Autodesk Inventor part; units mm, degrees
(part 3 of 4)
sketch "Эскиз8" plane through (0, 0, 5) normal (0, 0, 1) x (1, 0, 0)
  line L0 (-3.3401, -49.353) -> (-3.9955, -49.0011) projected
  line L1 (-3.9955, -49.0011) -> (-4.6711, -48.6896) projected
  line L2 (-4.6711, -48.6896) -> (-4.9594, -48.4736) projected
  line L3 (-4.9594, -48.4736) -> (-5.0531, -48.3399) projected
  line L4 (-5.0531, -48.3399) -> (-5.1131, -48.2201) projected
  line L5 (-5.1131, -48.2201) -> (-5.1548, -48.1078) projected
  line L6 (-5.1548, -48.1078) -> (-5.1842, -48.0004) projected
  line L7 (-5.1842, -48.0004) -> (-5.2179, -47.7953) projected
  line L8 (-5.2179, -47.7953) -> (-5.2276, -47.5993) projected
  line L9 (-5.2276, -47.5993) -> (-5.2195, -47.4096) projected
  line L10 (-5.2195, -47.4096) -> (-5.1972, -47.225) projected
  line L11 (-5.1972, -47.225) -> (-5.1181, -46.8673) projected
  line L12 (-5.1181, -46.8673) -> (-5.0105, -46.5192) projected
  line L13 (-5.0105, -46.5192) -> (-4.963, -46.1513) projected
  line L14 (-4.963, -46.1513) -> (-4.956, -45.7709) projected
  line L15 (-4.956, -45.7709) -> (-4.9802, -45.3817) projected
  line L16 (-4.9802, -45.3817) -> (-5.0317, -44.9857) projected
  line L17 (-5.0317, -44.9857) -> (-5.1086, -44.5842) projected
  line L18 (-5.1086, -44.5842) -> (-5.2096, -44.1783) projected
  line L19 (-5.2096, -44.1783) -> (-5.3339, -43.7691) projected
  line L20 (-5.3339, -43.7691) -> (-5.4808, -43.3575) projected
  line L21 (-5.4808, -43.3575) -> (-5.65, -42.9443) projected
  line L22 (-5.65, -42.9443) -> (-5.7913, -42.6339) projected
  line L23 (-5.7913, -42.6339) -> (-7.9172, -42.3165) projected
  line L24 (-7.9172, -42.3165) -> (-8.143, -42.5721) projected
  line L25 (-8.143, -42.5721) -> (-8.4255, -42.9179) projected
  line L26 (-8.4255, -42.9179) -> (-8.6862, -43.2687) projected
  line L27 (-8.6862, -43.2687) -> (-8.9246, -43.6237) projected
  line L28 (-8.9246, -43.6237) -> (-9.1398, -43.9824) projected
  line L29 (-9.1398, -43.9824) -> (-9.3306, -44.3439) projected
  line L30 (-9.3306, -44.3439) -> (-9.4955, -44.7076) projected
  line L31 (-9.4955, -44.7076) -> (-9.6323, -45.0728) projected
  line L32 (-9.6323, -45.0728) -> (-9.7367, -45.4387) projected
  line L33 (-9.7367, -45.4387) -> (-9.7987, -45.8044) projected
  line L34 (-9.7987, -45.8044) -> (-9.7975, -46.1687) projected
  line L35 (-9.7975, -46.1687) -> (-9.8263, -46.5339) projected
  line L36 (-9.8263, -46.5339) -> (-9.8589, -46.717) projected
  line L37 (-9.8589, -46.717) -> (-9.9066, -46.9008) projected
  line L38 (-9.9066, -46.9008) -> (-9.9731, -47.0854) projected
  line L39 (-9.9731, -47.0854) -> (-10.0652, -47.2717) projected
  line L40 (-10.0652, -47.2717) -> (-10.1248, -47.3659) projected
  line L41 (-10.1248, -47.3659) -> (-10.1974, -47.4611) projected
  line L42 (-10.1974, -47.4611) -> (-10.2897, -47.5581) projected
  line L43 (-10.2897, -47.5581) -> (-10.4185, -47.6586) projected
  line L44 (-10.4185, -47.6586) -> (-10.7573, -47.781) projected
  line L45 (-10.7573, -47.781) -> (-11.4943, -47.8816) projected
  line L46 (-11.4943, -47.8816) -> (-12.2239, -48.0267) projected
  line L47 (-12.2239, -48.0267) -> (-12.5841, -48.0214) projected
  line L48 (-12.5841, -48.0214) -> (-12.7386, -47.9683) projected
  line L49 (-12.7386, -47.9683) -> (-12.8575, -47.9067) projected
  line L50 (-12.8575, -47.9067) -> (-12.9572, -47.8403) projected
  line L51 (-12.9572, -47.8403) -> (-13.0442, -47.7707) projected
  line L52 (-13.0442, -47.7707) -> (-13.192, -47.6246) projected
  line L53 (-13.192, -47.6246) -> (-13.3151, -47.4717) projected
  line L54 (-13.3151, -47.4717) -> (-13.42, -47.3135) projected
  line L55 (-13.42, -47.3135) -> (-13.5105, -47.151) projected
  line L56 (-13.5105, -47.151) -> (-13.6567, -46.8152) projected
  line L57 (-13.6567, -46.8152) -> (-13.7743, -46.4703) projected
  line L58 (-13.7743, -46.4703) -> (-13.9521, -46.1448) projected
  line L59 (-13.9521, -46.1448) -> (-14.17, -45.8329) projected
  line L60 (-14.17, -45.8329) -> (-14.4183, -45.5322) projected
  line L61 (-14.4183, -45.5322) -> (-14.6928, -45.2421) projected
  line L62 (-14.6928, -45.2421) -> (-14.991, -44.9625) projected
  line L63 (-14.991, -44.9625) -> (-15.3113, -44.6935) projected
  line L64 (-15.3113, -44.6935) -> (-15.6524, -44.4355) projected
  line L65 (-15.6524, -44.4355) -> (-16.0132, -44.1889) projected
  line L66 (-16.0132, -44.1889) -> (-16.3929, -43.954) projected
  line L67 (-16.3929, -43.954) -> (-16.6897, -43.7859) projected
  line L68 (-16.6897, -43.7859) -> (-18.5962, -44.7788) projected
  line L69 (-18.5962, -44.7788) -> (-18.6286, -45.1183) projected
  line L70 (-18.6286, -45.1183) -> (-18.6538, -45.564) projected
  line L71 (-18.6538, -45.564) -> (-18.6586, -46.0011) projected
  line L72 (-18.6586, -46.0011) -> (-18.6428, -46.4284) projected
  line L73 (-18.6428, -46.4284) -> (-18.606, -46.8451) projected
  line L74 (-18.606, -46.8451) -> (-18.5479, -47.2497) projected
  line L75 (-18.5479, -47.2497) -> (-18.4676, -47.6409) projected
  line L76 (-18.4676, -47.6409) -> (-18.3636, -48.0168) projected
  line L77 (-18.3636, -48.0168) -> (-18.233, -48.3741) projected
  line L78 (-18.233, -48.3741) -> (-18.0682, -48.7064) projected
  line L79 (-18.0682, -48.7064) -> (-17.8531, -49.0005) projected
  line L80 (-17.8531, -49.0005) -> (-17.6617, -49.3128) projected
  line L81 (-17.6617, -49.3128) -> (-17.5804, -49.4801) projected
  line L82 (-17.5804, -49.4801) -> (-17.511, -49.6568) projected
  line L83 (-17.511, -49.6568) -> (-17.4563, -49.8453) projected
  line L84 (-17.4563, -49.8453) -> (-17.4213, -50.0502) projected
  line L85 (-17.4213, -50.0502) -> (-17.4142, -50.1613) projected
  line L86 (-17.4142, -50.1613) -> (-17.417, -50.2811) projected
  line L87 (-17.417, -50.2811) -> (-17.4346, -50.4138) projected
  line L88 (-17.4346, -50.4138) -> (-17.4797, -50.5708) projected
  line L89 (-17.4797, -50.5708) -> (-17.6818, -50.869) projected
  line L90 (-17.6818, -50.869) -> (-18.219, -51.3836) projected
  line L91 (-18.219, -51.3836) -> (-18.724, -51.9298) projected
  line L92 (-18.724, -51.9298) -> (-19.0185, -52.1372) projected
  line L93 (-19.0185, -52.1372) -> (-19.1747, -52.1851) projected
  line L94 (-19.1747, -52.1851) -> (-19.3071, -52.2051) projected
  line L95 (-19.3071, -52.2051) -> (-19.4268, -52.2101) projected
  line L96 (-19.4268, -52.2101) -> (-19.5381, -52.2049) projected
  line L97 (-19.5381, -52.2049) -> (-19.7435, -52.1736) projected
  line L98 (-19.7435, -52.1736) -> (-19.933, -52.1222) projected
  line L99 (-19.933, -52.1222) -> (-20.1108, -52.0559) projected
  line L100 (-20.1108, -52.0559) -> (-20.2796, -51.9776) projected
  line L101 (-20.2796, -51.9776) -> (-20.5952, -51.7918) projected
  line L102 (-20.5952, -51.7918) -> (-20.8931, -51.5819) projected
  line L103 (-20.8931, -51.5819) -> (-21.2283, -51.4231) projected
  line L104 (-21.2283, -51.4231) -> (-21.5879, -51.2989) projected
  line L105 (-21.5879, -51.2989) -> (-21.9655, -51.2016) projected
  line L106 (-21.9655, -51.2016) -> (-22.3581, -51.1282) projected
  line L107 (-22.3581, -51.1282) -> (-22.7637, -51.0773) projected
  line L108 (-22.7637, -51.0773) -> (-23.1809, -51.0479) projected
  line L109 (-23.1809, -51.0479) -> (-23.6085, -51.0397) projected
  line L110 (-23.6085, -51.0397) -> (-24.0454, -51.0522) projected
  line L111 (-24.0454, -51.0522) -> (-24.4906, -51.0855) projected
  line L112 (-24.4906, -51.0855) -> (-24.8295, -51.1239) projected
  line L113 (-24.8295, -51.1239) -> (-25.7883, -53.0477) projected
  line L114 (-25.7883, -53.0477) -> (-25.615, -53.3414) projected
  line L115 (-25.615, -53.3414) -> (-25.3734, -53.7169) projected
  line L116 (-25.3734, -53.7169) -> (-25.1204, -54.0733) projected
  line L117 (-25.1204, -54.0733) -> (-24.8564, -54.4097) projected
  line L118 (-24.8564, -54.4097) -> (-24.5818, -54.7252) projected
  line L119 (-24.5818, -54.7252) -> (-24.2969, -55.0184) projected
  line L120 (-24.2969, -55.0184) -> (-24.0019, -55.2877) projected
  line L121 (-24.0019, -55.2877) -> (-23.6969, -55.5306) projected
  line L122 (-23.6969, -55.5306) -> (-23.3812, -55.7429) projected
  line L123 (-23.3812, -55.7429) -> (-23.0526, -55.9149) projected
  line L124 (-23.0526, -55.9149) -> (-22.7057, -56.0264) projected
  line L125 (-22.7057, -56.0264) -> (-22.3673, -56.1666) projected
  line L126 (-22.3673, -56.1666) -> (-22.2032, -56.2542) projected
  line L127 (-22.2032, -56.2542) -> (-22.0432, -56.3563) projected
  line L128 (-22.0432, -56.3563) -> (-21.8881, -56.4766) projected
  line L129 (-21.8881, -56.4766) -> (-21.7394, -56.6218) projected
  line L130 (-21.7394, -56.6218) -> (-21.6683, -56.7075) projected
  line L131 (-21.6683, -56.7075) -> (-21.6001, -56.806) projected
  line L132 (-21.6001, -56.806) -> (-21.5364, -56.9238) projected
  line L133 (-21.5364, -56.9238) -> (-21.4806, -57.0773) projected
  line L134 (-21.4806, -57.0773) -> (-21.4689, -57.4374) projected
  line L135 (-21.4689, -57.4374) -> (-21.601, -58.1694) projected
  line L136 (-21.601, -58.1694) -> (-21.6884, -58.9082) projected
  line L137 (-21.6884, -58.9082) -> (-21.8048, -59.2491) projected
  line L138 (-21.8048, -59.2491) -> (-21.903, -59.3796) projected
  line L139 (-21.903, -59.3796) -> (-21.9984, -59.4736) projected
  line L140 (-21.9984, -59.4736) -> (-22.0923, -59.548) projected
  line L141 (-22.0923, -59.548) -> (-22.1854, -59.6092) projected
  line L142 (-22.1854, -59.6092) -> (-22.37, -59.7046) projected
  line L143 (-22.37, -59.7046) -> (-22.5535, -59.7744) projected
  line L144 (-22.5535, -59.7744) -> (-22.7363, -59.8253) projected
  line L145 (-22.7363, -59.8253) -> (-22.9189, -59.8611) projected
  line L146 (-22.9189, -59.8611) -> (-23.2834, -59.8964) projected
  line L147 (-23.2834, -59.8964) -> (-23.6478, -59.9017) projected
  line L148 (-23.6478, -59.9017) -> (-24.0123, -59.9702) projected
  line L149 (-24.0123, -59.9702) -> (-24.3762, -60.0811) projected
  line L150 (-24.3762, -60.0811) -> (-24.7389, -60.2243) projected
  line L151 (-24.7389, -60.2243) -> (-25.0997, -60.3957) projected
  line L152 (-25.0997, -60.3957) -> (-25.4578, -60.5929) projected
  line L153 (-25.4578, -60.5929) -> (-25.8125, -60.8144) projected
  line L154 (-25.8125, -60.8144) -> (-26.1633, -61.0591) projected
  line L155 (-26.1633, -61.0591) -> (-26.5094, -61.326) projected
  line L156 (-26.5094, -61.326) -> (-26.8501, -61.6146) projected
  line L157 (-26.8501, -61.6146) -> (-27.1017, -61.8449) projected
  line L158 (-27.1017, -61.8449) -> (-26.7465, -63.9648) projected
  line L159 (-26.7465, -63.9648) -> (-26.4337, -64.1006) projected
  line L160 (-26.4337, -64.1006) -> (-26.0175, -64.2624) projected
  line L161 (-26.0175, -64.2624) -> (-25.6033, -64.402) projected
  line L162 (-25.6033, -64.402) -> (-25.192, -64.519) projected
  line L163 (-25.192, -64.519) -> (-24.7844, -64.6128) projected
  line L164 (-24.7844, -64.6128) -> (-24.3816, -64.6825) projected
  line L165 (-24.3816, -64.6825) -> (-23.9847, -64.727) projected
  line L166 (-23.9847, -64.727) -> (-23.5951, -64.7442) projected
  line L167 (-23.5951, -64.7442) -> (-23.2149, -64.7305) projected
  line L168 (-23.2149, -64.7305) -> (-22.848, -64.6765) projected
  line L169 (-22.848, -64.6765) -> (-22.5018, -64.5627) projected
  line L170 (-22.5018, -64.5627) -> (-22.1456, -64.4773) projected
  line L171 (-22.1456, -64.4773) -> (-21.9614, -64.4516) projected
  line L172 (-21.9614, -64.4516) -> (-21.7719, -64.4402) projected
  line L173 (-21.7719, -64.4402) -> (-21.5757, -64.4464) projected
  line L174 (-21.5757, -64.4464) -> (-21.3701, -64.4764) projected
  line L175 (-21.3701, -64.4764) -> (-21.2621, -64.504) projected
  line L176 (-21.2621, -64.504) -> (-21.1491, -64.5437) projected
  line L177 (-21.1491, -64.5437) -> (-21.0284, -64.6015) projected
  line L178 (-21.0284, -64.6015) -> (-20.8929, -64.6929) projected
  line L179 (-20.8929, -64.6929) -> (-20.6718, -64.9773) projected
  line L180 (-20.6718, -64.9773) -> (-20.3484, -65.6472) projected
  line L181 (-20.3484, -65.6472) -> (-19.985, -66.2962) projected
  circle A0 centre (-9.4677, -59.9808) radius 2.5 projected
  circle A1 centre (-2.274, -63.481) radius 1.6 projected
  circle A2 centre (-5.9675, -52.7871) radius 1.6 projected
  circle A3 centre (-16.6613, -56.4807) radius 1.6 projected
  circle A4 centre (-12.9678, -67.1745) radius 1.6 projected
  arc A5 (-27.2901, -112.9599) -> (-22.8404, -113.0615) centre (-25.0135, -110.7468) ccw projected
  line L182 (-25.0135, -110.7468) -> (-25.0135, -76.7468)
  line L183 (-25.0135, -110.7468) -> (8.9865, -110.7468) construction
  line L184 (-46.2049, -99.4426) -> (-29.9022, -115.8548)
  line L185 (-29.9022, -115.8548) -> (-56.6455, -115.6472)
  line L186 (-25.5981, -48.7632) -> (-26.9625, -47.1023) projected
  line L187 (-27.3014, -47.1406) -> (-26.9625, -47.1023) projected
  line L188 (-27.7429, -47.2077) -> (-27.3014, -47.1406) projected
  line L189 (-28.1715, -47.2931) -> (-27.7429, -47.2077) projected
  line L190 (-28.5864, -47.3967) -> (-28.1715, -47.2931) projected
  line L191 (-28.9865, -47.5185) -> (-28.5864, -47.3967) projected
  line L192 (-29.3705, -47.6588) -> (-28.9865, -47.5185) projected
  line L193 (-29.7368, -47.818) -> (-29.3705, -47.6588) projected
  line L194 (-30.0831, -47.9973) -> (-29.7368, -47.818) projected
  line L195 (-30.4059, -48.1987) -> (-30.0831, -47.9973) projected
  line L196 (-30.6971, -48.4284) -> (-30.4059, -48.1987) projected
  line L197 (-30.9405, -48.6995) -> (-30.6971, -48.4284) projected
  line L198 (-31.2067, -48.9511) -> (-30.9405, -48.6995) projected
  line L199 (-31.3536, -49.0652) -> (-31.2067, -48.9511) projected
  line L200 (-31.5122, -49.1695) -> (-31.3536, -49.0652) projected
  line L201 (-31.6854, -49.262) -> (-31.5122, -49.1695) projected
  line L202 (-31.8786, -49.3384) -> (-31.6854, -49.262) projected
  line L203 (-31.986, -49.3683) -> (-31.8786, -49.3384) projected
  line L204 (-32.1037, -49.3902) -> (-31.986, -49.3683) projected
  line L205 (-32.2372, -49.4003) -> (-32.1037, -49.3902) projected
  line L206 (-32.4002, -49.3886) -> (-32.2372, -49.4003) projected
  line L207 (-32.7336, -49.2522) -> (-32.4002, -49.3886) projected
  line L208 (-33.3479, -48.8326) -> (-32.7336, -49.2522) projected
  line L209 (-33.9864, -48.4511) -> (-33.3479, -48.8326) projected
  line L210 (-34.2501, -48.2056) -> (-33.9864, -48.4511) projected
  line L211 (-34.3291, -48.0626) -> (-34.2501, -48.2056) projected
  line L212 (-34.376, -47.9372) -> (-34.3291, -48.0626) projected
  line L213 (-34.4055, -47.8211) -> (-34.376, -47.9372) projected
  line L214 (-34.4234, -47.7112) -> (-34.4055, -47.8211) projected
  line L215 (-34.4351, -47.5037) -> (-34.4234, -47.7112) projected
  line L216 (-34.4238, -47.3077) -> (-34.4351, -47.5037) projected
  line L217 (-34.3956, -47.12) -> (-34.4238, -47.3077) projected
  line L218 (-34.3538, -46.9387) -> (-34.3956, -47.12) projected
  line L219 (-34.237, -46.5916) -> (-34.3538, -46.9387) projected
  line L220 (-34.0931, -46.2568) -> (-34.237, -46.5916) projected
  line L221 (-34.0067, -45.8961) -> (-34.0931, -46.2568) projected
  line L222 (-33.9593, -45.5186) -> (-34.0067, -45.8961) projected
  line L223 (-33.9419, -45.129) -> (-33.9593, -45.5186) projected
  line L224 (-33.951, -44.7298) -> (-33.9419, -45.129) projected
  line L225 (-33.9848, -44.3224) -> (-33.951, -44.7298) projected
  line L226 (-34.0421, -43.9081) -> (-33.9848, -44.3224) projected
  line L227 (-34.1221, -43.488) -> (-34.0421, -43.9081) projected
  line L228 (-34.2244, -43.063) -> (-34.1221, -43.488) projected
  line L229 (-34.3487, -42.6342) -> (-34.2244, -43.063) projected
  line L230 (-34.4561, -42.3105) -> (-34.3487, -42.6342) projected
  line L231 (-36.5363, -41.7688) -> (-34.4561, -42.3105) projected
  line L232 (-36.7879, -41.999) -> (-36.5363, -41.7688) projected
  line L233 (-37.1056, -42.3127) -> (-36.7879, -41.999) projected
  line L234 (-37.4022, -42.6338) -> (-37.1056, -42.3127) projected
  line L235 (-37.677, -42.9614) -> (-37.4022, -42.6338) projected
  line L236 (-37.9291, -43.2952) -> (-37.677, -42.9614) projected
  line L237 (-38.1573, -43.6344) -> (-37.9291, -43.2952) projected
  line L238 (-38.36, -43.9785) -> (-38.1573, -43.6344) projected
  line L239 (-38.5348, -44.327) -> (-38.36, -43.9785) projected
  line L240 (-38.6775, -44.6797) -> (-38.5348, -44.327) projected
  line L241 (-38.7781, -45.0367) -> (-38.6775, -44.6797) projected
  line L242 (-38.8157, -45.3992) -> (-38.7781, -45.0367) projected
  line L243 (-38.8831, -45.7592) -> (-38.8157, -45.3992) projected
  line L244 (-38.935, -45.9378) -> (-38.8831, -45.7592) projected
  line L245 (-39.0019, -46.1155) -> (-38.935, -45.9378) projected
  line L246 (-39.0877, -46.292) -> (-39.0019, -46.1155) projected
  line L247 (-39.1991, -46.4674) -> (-39.0877, -46.292) projected
  line L248 (-39.2684, -46.5547) -> (-39.1991, -46.4674) projected
  line L249 (-39.3507, -46.6417) -> (-39.2684, -46.5547) projected
  line L250 (-39.4528, -46.7283) -> (-39.3507, -46.6417) projected
  line L251 (-39.5916, -46.8146) -> (-39.4528, -46.7283) projected
  line L252 (-39.9414, -46.9002) -> (-39.5916, -46.8146) projected
  line L253 (-40.685, -46.9219) -> (-39.9414, -46.9002) projected
  line L254 (-41.4259, -46.9885) -> (-40.685, -46.9219) projected
  line L255 (-41.7835, -46.9449) -> (-41.4259, -46.9885) projected
  line L256 (-41.9315, -46.8757) -> (-41.7835, -46.9449) projected
  line L257 (-42.0431, -46.8018) -> (-41.9315, -46.8757) projected
  line L258 (-42.1352, -46.7252) -> (-42.0431, -46.8018) projected
  line L259 (-42.2143, -46.6467) -> (-42.1352, -46.7252) projected
  line L260 (-42.3457, -46.4857) -> (-42.2143, -46.6467) projected
  line L261 (-42.4518, -46.3206) -> (-42.3457, -46.4857) projected
  line L262 (-42.5394, -46.1522) -> (-42.4518, -46.3206) projected
  line L263 (-42.612, -45.9809) -> (-42.5394, -46.1522) projected
  line L264 (-42.7217, -45.6314) -> (-42.612, -45.9809) projected
  line L265 (-42.8019, -45.276) -> (-42.7217, -45.6314) projected
  line L266 (-42.9441, -44.9334) -> (-42.8019, -45.276) projected
  line L267 (-43.1276, -44.6002) -> (-42.9441, -44.9334) projected
  line L268 (-43.3425, -44.2748) -> (-43.1276, -44.6002) projected
  line L269 (-43.5846, -43.9571) -> (-43.3425, -44.2748) projected
  line L270 (-43.8514, -43.6473) -> (-43.5846, -43.9571) projected
  line L271 (-44.1412, -43.3458) -> (-43.8514, -43.6473) projected
  line L272 (-44.4529, -43.053) -> (-44.1412, -43.3458) projected
  line L273 (-44.5941, -42.9326) -> (-44.4529, -43.053) projected
  arc A6 (-44.5941, -42.9326) -> (-50.5827, -73.1948) centre (-31.1137, -61.3239) ccw projected
  arc A7 (-46.3063, -82.796) -> (-50.5827, -73.1948) centre (-85.5886, -94.5392) ccw projected
  line L274 (-46.3063, -82.796) -> (-63.0717, -107.6742) projected
  line L275 (-63.0717, -107.6742) -> (-48.9946, -134.1664) projected
  line L276 (-48.9946, -134.1664) -> (-45.4623, -132.2894) projected
  line L277 (-45.4623, -132.2894) -> (-58.0098, -108.6759) projected
  line L278 (-58.0098, -108.6759) -> (-41.2444, -83.7977) projected
  line L279 (-26.1708, -65.5638) -> (-41.2444, -83.7977) projected
  line L280 (-26.1708, -65.5638) -> (-26.1132, -65.2728) projected
  line L281 (-26.2817, -65.1065) -> (-26.1132, -65.2728) projected
  line L282 (-26.573, -64.8618) -> (-26.2817, -65.1065) projected
  line L283 (-26.8814, -64.6558) -> (-26.573, -64.8618) projected
  line L284 (-27.2145, -64.5081) -> (-26.8814, -64.6558) projected
  line L285 (-27.5361, -64.3327) -> (-27.2145, -64.5081) projected
  line L286 (-27.6899, -64.2282) -> (-27.5361, -64.3327) projected
  line L287 (-27.8382, -64.1096) -> (-27.6899, -64.2282) projected
  line L288 (-27.9796, -63.9735) -> (-27.8382, -64.1096) projected
  line L289 (-28.112, -63.8133) -> (-27.9796, -63.9735) projected
  line L290 (-28.1736, -63.7205) -> (-28.112, -63.8133) projected
  line L291 (-28.2309, -63.6153) -> (-28.1736, -63.7205) projected
  line L292 (-28.2817, -63.4914) -> (-28.2309, -63.6153) projected
  line L293 (-28.3209, -63.3328) -> (-28.2817, -63.4914) projected
  line L294 (-28.2942, -62.9735) -> (-28.3209, -63.3328) projected
  line L295 (-28.085, -62.2597) -> (-28.2942, -62.9735) projected
  line L296 (-27.9195, -61.5344) -> (-28.085, -62.2597) projected
  line L297 (-27.7675, -61.2078) -> (-27.9195, -61.5344) projected
  line L298 (-27.6559, -61.0885) -> (-27.7675, -61.2078) projected
  line L299 (-27.5511, -61.0052) -> (-27.6559, -61.0885) projected
  line L300 (-27.4498, -60.9413) -> (-27.5511, -61.0052) projected
  line L301 (-27.3508, -60.8903) -> (-27.4498, -60.9413) projected
  line L302 (-27.1571, -60.815) -> (-27.3508, -60.8903) projected
  line L303 (-26.9672, -60.7651) -> (-27.1571, -60.815) projected
  line L304 (-26.78, -60.734) -> (-26.9672, -60.7651) projected
  line L305 (-26.5947, -60.7178) -> (-26.78, -60.734) projected
  line L306 (-26.2284, -60.7215) -> (-26.5947, -60.7178) projected
  line L307 (-25.8656, -60.755) -> (-26.2284, -60.7215) projected
  line L308 (-25.4958, -60.7256) -> (-25.8656, -60.755) projected
  line L309 (-25.1221, -60.6541) -> (-25.4958, -60.7256) projected
  line L310 (-24.7463, -60.5502) -> (-25.1221, -60.6541) projected
  line L311 (-24.3693, -60.4182) -> (-24.7463, -60.5502) projected
  line L312 (-23.9923, -60.2602) -> (-24.3693, -60.4182) projected
  line L313 (-23.616, -60.0777) -> (-23.9923, -60.2602) projected
  line L314 (-23.2412, -59.8717) -> (-23.616, -60.0777) projected
  line L315 (-22.8687, -59.6431) -> (-23.2412, -59.8717) projected
  line L316 (-22.4992, -59.3924) -> (-22.8687, -59.6431) projected
  line L317 (-22.2246, -59.1902) -> (-22.4992, -59.3924) projected
  line L318 (-22.3522, -57.0445) -> (-22.2246, -59.1902) projected
  line L319 (-22.6489, -56.8763) -> (-22.3522, -57.0445) projected
  line L320 (-23.0454, -56.6711) -> (-22.6489, -56.8763) projected
  line L321 (-23.4424, -56.4882) -> (-23.0454, -56.6711) projected
  line L322 (-23.839, -56.3281) -> (-23.4424, -56.4882) projected
  line L323 (-24.2343, -56.1915) -> (-23.839, -56.3281) projected
  line L324 (-24.6274, -56.0793) -> (-24.2343, -56.1915) projected
  line L325 (-25.0173, -55.9929) -> (-24.6274, -56.0793) projected
  line L326 (-25.4028, -55.9343) -> (-25.0173, -55.9929) projected
  line L327 (-25.7823, -55.9075) -> (-25.4028, -55.9343) projected
  line L328 (-26.153, -55.9222) -> (-25.7823, -55.9075) projected
  line L329 (-26.5093, -55.9985) -> (-26.153, -55.9222) projected
  line L330 (-26.8725, -56.0456) -> (-26.5093, -55.9985) projected
  line L331 (-27.0584, -56.0515) -> (-26.8725, -56.0456) projected
  line L332 (-27.248, -56.0427) -> (-27.0584, -56.0515) projected
  line L333 (-27.4425, -56.0157) -> (-27.248, -56.0427) projected
  line L334 (-27.6437, -55.9639) -> (-27.4425, -56.0157) projected
  line L335 (-27.7481, -55.925) -> (-27.6437, -55.9639) projected
  line L336 (-27.8563, -55.8736) -> (-27.7481, -55.925) projected
  line L337 (-27.9702, -55.8032) -> (-27.8563, -55.8736) projected
  line L338 (-28.0951, -55.698) -> (-27.9702, -55.8032) projected
  line L339 (-28.2847, -55.3917) -> (-28.0951, -55.698) projected
  line L340 (-28.5351, -54.6912) -> (-28.2847, -55.3917) projected
  line L341 (-28.8274, -54.0071) -> (-28.5351, -54.6912) projected
  line L342 (-28.8965, -53.6536) -> (-28.8274, -54.0071) projected
  line L343 (-28.8763, -53.4914) -> (-28.8965, -53.6536) projected
  line L344 (-28.8405, -53.3624) -> (-28.8763, -53.4914) projected
  line L345 (-28.7962, -53.2512) -> (-28.8405, -53.3624) projected
  line L346 (-28.746, -53.1517) -> (-28.7962, -53.2512) projected
  line L347 (-28.6335, -52.977) -> (-28.746, -53.1517) projected
  line L348 (-28.5092, -52.825) -> (-28.6335, -52.977) projected
  line L349 (-28.3761, -52.6897) -> (-28.5092, -52.825) projected
  line L350 (-28.2357, -52.5677) -> (-28.3761, -52.6897) projected
  line L351 (-27.9372, -52.3554) -> (-28.2357, -52.5677) projected
  line L352 (-27.624, -52.1693) -> (-27.9372, -52.3554) projected
  line L353 (-27.3421, -51.9282) -> (-27.624, -52.1693) projected
  line L354 (-27.0818, -51.6507) -> (-27.3421, -51.9282) projected
  line L355 (-26.8388, -51.3457) -> (-27.0818, -51.6507) projected
  line L356 (-26.6114, -51.0173) -> (-26.8388, -51.3457) projected
  line L357 (-26.3993, -50.6679) -> (-26.6114, -51.0173) projected
  line L358 (-26.2021, -50.2991) -> (-26.3993, -50.6679) projected
  line L359 (-26.02, -49.9121) -> (-26.2021, -50.2991) projected
  line L360 (-25.853, -49.5082) -> (-26.02, -49.9121) projected
  line L361 (-25.7014, -49.0882) -> (-25.853, -49.5082) projected
  line L362 (-25.5981, -48.7632) -> (-25.7014, -49.0882) projected
  circle A8 centre (-42.8052, -51.6922) radius 1.6 projected
  circle A9 centre (-39.9568, -59.168) radius 2.5 projected
  circle A10 centre (-32.4811, -56.3196) radius 1.6 projected
  circle A11 centre (-37.1084, -66.6437) radius 1.6 projected
  circle A12 centre (-47.4326, -62.0164) radius 1.6 projected
  line L363 (-46.3063, -82.796) -> (-41.3132, -83.8997)
  line L364 (-46.2049, -99.4426) -> (-41.3132, -83.8997)
  line L365 (-46.3063, -82.796) -> (-56.6455, -115.6472)
  arc A13 (-19.985, -66.2962) -> (-3.3401, -49.353) centre (-9.4677, -59.9808) ccw projected
  point P0 (0, 0)
  point P1 (-42.8913, -102.7785)
  point P2 (-56.6509, -115.6472)
  point P3 (-55.7751, -112.8815)
  point P4 (-54.2957, -115.6655)
  dimension "d21" = 34
  dimension "d22" = 90
  constraints: 14 end point, 3 point on line, 1 horizontal, 1 parallel, 1 perpendicular, 1 vertical
  measures "d21" distance of L182.start L182.end
  measures "d22" angle of L183 L182
extrude "Выдавливание8" add sketch "Эскиз8" against normal up to surface (5 mm away) contours L364 L184 L185 L277 L365 L278 | L278 L365 L363
sketch "Эскиз9" plane through (0, 0, 5) normal (0, 0, 1) x (1, 0, 0)
  line L0 (-41.3132, -83.8997) -> (-41.2444, -83.7977) projected
  line L1 (-26.1708, -65.5638) -> (-41.2444, -83.7977) projected
  line L2 (-26.1708, -65.5638) -> (-26.1132, -65.2728) projected
  line L3 (-26.2817, -65.1065) -> (-26.1132, -65.2728) projected
  line L4 (-26.573, -64.8618) -> (-26.2817, -65.1065) projected
  line L5 (-26.8814, -64.6558) -> (-26.573, -64.8618) projected
  line L6 (-27.2145, -64.5081) -> (-26.8814, -64.6558) projected
  line L7 (-27.5361, -64.3327) -> (-27.2145, -64.5081) projected
  line L8 (-27.6899, -64.2282) -> (-27.5361, -64.3327) projected
  line L9 (-27.8382, -64.1096) -> (-27.6899, -64.2282) projected
  line L10 (-27.9796, -63.9735) -> (-27.8382, -64.1096) projected
  line L11 (-28.112, -63.8133) -> (-27.9796, -63.9735) projected
  line L12 (-28.1736, -63.7205) -> (-28.112, -63.8133) projected
  line L13 (-28.2309, -63.6153) -> (-28.1736, -63.7205) projected
  line L14 (-28.2817, -63.4914) -> (-28.2309, -63.6153) projected
  line L15 (-28.3209, -63.3328) -> (-28.2817, -63.4914) projected
  line L16 (-28.2942, -62.9735) -> (-28.3209, -63.3328) projected
  line L17 (-28.085, -62.2597) -> (-28.2942, -62.9735) projected
  line L18 (-27.9195, -61.5344) -> (-28.085, -62.2597) projected
  line L19 (-27.7675, -61.2078) -> (-27.9195, -61.5344) projected
  line L20 (-27.6559, -61.0885) -> (-27.7675, -61.2078) projected
  line L21 (-27.5511, -61.0052) -> (-27.6559, -61.0885) projected
  line L22 (-27.4498, -60.9413) -> (-27.5511, -61.0052) projected
  line L23 (-27.3508, -60.8903) -> (-27.4498, -60.9413) projected
  line L24 (-27.1571, -60.815) -> (-27.3508, -60.8903) projected
  line L25 (-26.9672, -60.7651) -> (-27.1571, -60.815) projected
  line L26 (-26.78, -60.734) -> (-26.9672, -60.7651) projected
  line L27 (-26.5947, -60.7178) -> (-26.78, -60.734) projected
  line L28 (-26.2284, -60.7215) -> (-26.5947, -60.7178) projected
  line L29 (-25.8656, -60.755) -> (-26.2284, -60.7215) projected
  line L30 (-25.4958, -60.7256) -> (-25.8656, -60.755) projected
  line L31 (-25.1221, -60.6541) -> (-25.4958, -60.7256) projected
  line L32 (-24.7463, -60.5502) -> (-25.1221, -60.6541) projected
  line L33 (-24.3693, -60.4182) -> (-24.7463, -60.5502) projected
  line L34 (-23.9923, -60.2602) -> (-24.3693, -60.4182) projected
  line L35 (-23.616, -60.0777) -> (-23.9923, -60.2602) projected
  line L36 (-23.2412, -59.8717) -> (-23.616, -60.0777) projected
  line L37 (-22.8687, -59.6431) -> (-23.2412, -59.8717) projected
  line L38 (-22.4992, -59.3924) -> (-22.8687, -59.6431) projected
  line L39 (-22.2246, -59.1902) -> (-22.4992, -59.3924) projected
  line L40 (-22.3522, -57.0445) -> (-22.2246, -59.1902) projected
  line L41 (-22.6489, -56.8763) -> (-22.3522, -57.0445) projected
  line L42 (-23.0454, -56.6711) -> (-22.6489, -56.8763) projected
  line L43 (-23.4424, -56.4882) -> (-23.0454, -56.6711) projected
  line L44 (-23.839, -56.3281) -> (-23.4424, -56.4882) projected
  line L45 (-24.2343, -56.1915) -> (-23.839, -56.3281) projected
  line L46 (-24.6274, -56.0793) -> (-24.2343, -56.1915) projected
  line L47 (-25.0173, -55.9929) -> (-24.6274, -56.0793) projected
  line L48 (-25.4028, -55.9343) -> (-25.0173, -55.9929) projected
  line L49 (-25.7823, -55.9075) -> (-25.4028, -55.9343) projected
  line L50 (-26.153, -55.9222) -> (-25.7823, -55.9075) projected
  line L51 (-26.5093, -55.9985) -> (-26.153, -55.9222) projected
  line L52 (-26.8725, -56.0456) -> (-26.5093, -55.9985) projected
  line L53 (-27.0584, -56.0515) -> (-26.8725, -56.0456) projected
  line L54 (-27.248, -56.0427) -> (-27.0584, -56.0515) projected
  line L55 (-27.4425, -56.0157) -> (-27.248, -56.0427) projected
  line L56 (-27.6437, -55.9639) -> (-27.4425, -56.0157) projected
  line L57 (-27.7481, -55.925) -> (-27.6437, -55.9639) projected
  line L58 (-27.8563, -55.8736) -> (-27.7481, -55.925) projected
  line L59 (-27.9702, -55.8032) -> (-27.8563, -55.8736) projected
  line L60 (-28.0951, -55.698) -> (-27.9702, -55.8032) projected
  line L61 (-28.2847, -55.3917) -> (-28.0951, -55.698) projected
  line L62 (-28.5351, -54.6912) -> (-28.2847, -55.3917) projected
  line L63 (-28.8274, -54.0071) -> (-28.5351, -54.6912) projected
  line L64 (-28.8965, -53.6536) -> (-28.8274, -54.0071) projected
  line L65 (-28.8763, -53.4914) -> (-28.8965, -53.6536) projected
  line L66 (-28.8405, -53.3624) -> (-28.8763, -53.4914) projected
  line L67 (-28.7962, -53.2512) -> (-28.8405, -53.3624) projected
  line L68 (-28.746, -53.1517) -> (-28.7962, -53.2512) projected
  line L69 (-28.6335, -52.977) -> (-28.746, -53.1517) projected
  line L70 (-28.5092, -52.825) -> (-28.6335, -52.977) projected
  line L71 (-28.3761, -52.6897) -> (-28.5092, -52.825) projected
  line L72 (-28.2357, -52.5677) -> (-28.3761, -52.6897) projected
  line L73 (-27.9372, -52.3554) -> (-28.2357, -52.5677) projected
  line L74 (-27.624, -52.1693) -> (-27.9372, -52.3554) projected
  line L75 (-27.3421, -51.9282) -> (-27.624, -52.1693) projected
  line L76 (-27.0818, -51.6507) -> (-27.3421, -51.9282) projected
  line L77 (-26.8388, -51.3457) -> (-27.0818, -51.6507) projected
  line L78 (-26.6114, -51.0173) -> (-26.8388, -51.3457) projected
  line L79 (-26.3993, -50.6679) -> (-26.6114, -51.0173) projected
  line L80 (-26.2021, -50.2991) -> (-26.3993, -50.6679) projected
  line L81 (-26.02, -49.9121) -> (-26.2021, -50.2991) projected
  line L82 (-25.853, -49.5082) -> (-26.02, -49.9121) projected
  line L83 (-25.7014, -49.0882) -> (-25.853, -49.5082) projected
  line L84 (-25.5981, -48.7632) -> (-25.7014, -49.0882) projected
  line L85 (-25.5981, -48.7632) -> (-26.9625, -47.1023) projected
  line L86 (-27.3014, -47.1406) -> (-26.9625, -47.1023) projected
  line L87 (-27.7429, -47.2077) -> (-27.3014, -47.1406) projected
  line L88 (-28.1715, -47.2931) -> (-27.7429, -47.2077) projected
  line L89 (-28.5864, -47.3967) -> (-28.1715, -47.2931) projected
  line L90 (-28.9865, -47.5185) -> (-28.5864, -47.3967) projected
  line L91 (-29.3705, -47.6588) -> (-28.9865, -47.5185) projected
  line L92 (-29.7368, -47.818) -> (-29.3705, -47.6588) projected
  line L93 (-30.0831, -47.9973) -> (-29.7368, -47.818) projected
  line L94 (-30.4059, -48.1987) -> (-30.0831, -47.9973) projected
  line L95 (-30.6971, -48.4284) -> (-30.4059, -48.1987) projected
  line L96 (-30.9405, -48.6995) -> (-30.6971, -48.4284) projected
  line L97 (-31.2067, -48.9511) -> (-30.9405, -48.6995) projected
  line L98 (-31.3536, -49.0652) -> (-31.2067, -48.9511) projected
  line L99 (-31.5122, -49.1695) -> (-31.3536, -49.0652) projected
  line L100 (-31.6854, -49.262) -> (-31.5122, -49.1695) projected
  line L101 (-31.8786, -49.3384) -> (-31.6854, -49.262) projected
  line L102 (-31.986, -49.3683) -> (-31.8786, -49.3384) projected
  line L103 (-32.1037, -49.3902) -> (-31.986, -49.3683) projected
  line L104 (-32.2372, -49.4003) -> (-32.1037, -49.3902) projected
  line L105 (-32.4002, -49.3886) -> (-32.2372, -49.4003) projected
  line L106 (-32.7336, -49.2522) -> (-32.4002, -49.3886) projected
  line L107 (-33.3479, -48.8326) -> (-32.7336, -49.2522) projected
  line L108 (-33.9864, -48.4511) -> (-33.3479, -48.8326) projected
  line L109 (-34.2501, -48.2056) -> (-33.9864, -48.4511) projected
  line L110 (-34.3291, -48.0626) -> (-34.2501, -48.2056) projected
  line L111 (-34.376, -47.9372) -> (-34.3291, -48.0626) projected
  line L112 (-34.4055, -47.8211) -> (-34.376, -47.9372) projected
  line L113 (-34.4234, -47.7112) -> (-34.4055, -47.8211) projected
  line L114 (-34.4351, -47.5037) -> (-34.4234, -47.7112) projected
  line L115 (-34.4238, -47.3077) -> (-34.4351, -47.5037) projected
  line L116 (-34.3956, -47.12) -> (-34.4238, -47.3077) projected
  line L117 (-34.3538, -46.9387) -> (-34.3956, -47.12) projected
  line L118 (-34.237, -46.5916) -> (-34.3538, -46.9387) projected
  line L119 (-34.0931, -46.2568) -> (-34.237, -46.5916) projected
  line L120 (-34.0067, -45.8961) -> (-34.0931, -46.2568) projected
  line L121 (-33.9593, -45.5186) -> (-34.0067, -45.8961) projected
  line L122 (-33.9419, -45.129) -> (-33.9593, -45.5186) projected
  line L123 (-33.951, -44.7298) -> (-33.9419, -45.129) projected
  line L124 (-33.9848, -44.3224) -> (-33.951, -44.7298) projected
  line L125 (-34.0421, -43.9081) -> (-33.9848, -44.3224) projected
  line L126 (-34.1221, -43.488) -> (-34.0421, -43.9081) projected
  line L127 (-34.2244, -43.063) -> (-34.1221, -43.488) projected
  line L128 (-34.3487, -42.6342) -> (-34.2244, -43.063) projected
  line L129 (-34.4561, -42.3105) -> (-34.3487, -42.6342) projected
  line L130 (-36.5363, -41.7688) -> (-34.4561, -42.3105) projected
  line L131 (-36.7879, -41.999) -> (-36.5363, -41.7688) projected
  line L132 (-37.1056, -42.3127) -> (-36.7879, -41.999) projected
  line L133 (-37.4022, -42.6338) -> (-37.1056, -42.3127) projected
  line L134 (-37.677, -42.9614) -> (-37.4022, -42.6338) projected
  line L135 (-37.9291, -43.2952) -> (-37.677, -42.9614) projected
  line L136 (-38.1573, -43.6344) -> (-37.9291, -43.2952) projected
  line L137 (-38.36, -43.9785) -> (-38.1573, -43.6344) projected
  line L138 (-38.5348, -44.327) -> (-38.36, -43.9785) projected
  line L139 (-38.6775, -44.6797) -> (-38.5348, -44.327) projected
  line L140 (-38.7781, -45.0367) -> (-38.6775, -44.6797) projected
  line L141 (-38.8157, -45.3992) -> (-38.7781, -45.0367) projected
  line L142 (-38.8831, -45.7592) -> (-38.8157, -45.3992) projected
  line L143 (-38.935, -45.9378) -> (-38.8831, -45.7592) projected
  line L144 (-39.0019, -46.1155) -> (-38.935, -45.9378) projected
  line L145 (-39.0877, -46.292) -> (-39.0019, -46.1155) projected
  line L146 (-39.1991, -46.4674) -> (-39.0877, -46.292) projected
  line L147 (-39.2684, -46.5547) -> (-39.1991, -46.4674) projected
  line L148 (-39.3507, -46.6417) -> (-39.2684, -46.5547) projected
  line L149 (-39.4528, -46.7283) -> (-39.3507, -46.6417) projected
  line L150 (-39.5916, -46.8146) -> (-39.4528, -46.7283) projected
  line L151 (-39.9414, -46.9002) -> (-39.5916, -46.8146) projected
  line L152 (-40.685, -46.9219) -> (-39.9414, -46.9002) projected
  line L153 (-41.4259, -46.9885) -> (-40.685, -46.9219) projected
  line L154 (-41.7835, -46.9449) -> (-41.4259, -46.9885) projected
  line L155 (-41.9315, -46.8757) -> (-41.7835, -46.9449) projected
  line L156 (-42.0431, -46.8018) -> (-41.9315, -46.8757) projected
  line L157 (-42.1352, -46.7252) -> (-42.0431, -46.8018) projected
  line L158 (-42.2143, -46.6467) -> (-42.1352, -46.7252) projected
  line L159 (-42.3457, -46.4857) -> (-42.2143, -46.6467) projected
  line L160 (-42.4518, -46.3206) -> (-42.3457, -46.4857) projected
  line L161 (-42.5394, -46.1522) -> (-42.4518, -46.3206) projected
  line L162 (-42.612, -45.9809) -> (-42.5394, -46.1522) projected
  line L163 (-42.7217, -45.6314) -> (-42.612, -45.9809) projected
  line L164 (-42.8019, -45.276) -> (-42.7217, -45.6314) projected
  line L165 (-42.9441, -44.9334) -> (-42.8019, -45.276) projected
  line L166 (-43.1276, -44.6002) -> (-42.9441, -44.9334) projected
  line L167 (-43.3425, -44.2748) -> (-43.1276, -44.6002) projected
  line L168 (-43.5846, -43.9571) -> (-43.3425, -44.2748) projected
  line L169 (-43.8514, -43.6473) -> (-43.5846, -43.9571) projected
  line L170 (-44.1412, -43.3458) -> (-43.8514, -43.6473) projected
  line L171 (-44.4529, -43.053) -> (-44.1412, -43.3458) projected
  line L172 (-44.5941, -42.9326) -> (-44.4529, -43.053) projected
  arc A0 (-44.5941, -42.9326) -> (-50.5827, -73.1948) centre (-31.1137, -61.3239) ccw projected
  arc A1 (-46.3063, -82.796) -> (-50.5827, -73.1948) centre (-85.5886, -94.5392) ccw projected
  line L173 (-46.3063, -82.796) -> (-63.0717, -107.6742) projected
  line L174 (-63.0717, -107.6742) -> (-48.9946, -134.1664) projected
  line L175 (-48.9946, -134.1664) -> (-45.4623, -132.2894) projected
  line L176 (-45.4623, -132.2894) -> (-54.2957, -115.6655) projected
  line L177 (-54.2957, -115.6655) -> (-29.9022, -115.8548) projected
  line L178 (-29.9022, -115.8548) -> (-46.2049, -99.4426) projected
  line L179 (-46.2049, -99.4426) -> (-41.3132, -83.8997) projected
  circle A2 centre (-47.4326, -62.0164) radius 1.6 projected
  circle A3 centre (-37.1084, -66.6437) radius 1.6 projected
  circle A4 centre (-32.4811, -56.3196) radius 1.6 projected
  circle A5 centre (-39.9568, -59.168) radius 2.5 projected
  circle A6 centre (-42.8052, -51.6922) radius 1.6 projected
  line L180 (-51.3334, -98.7688) -> (-55.7751, -112.8815) projected
  line L181 (-55.7751, -112.8815) -> (-58.0098, -108.6759) projected
  line L182 (-58.0098, -108.6759) -> (-51.3334, -98.7688) projected
  line L183 (-51.3334, -98.7688) -> (-46.3063, -82.796)
  line L184 (-55.7751, -112.8815) -> (-55.7748, -115.6656)
  line L185 (-55.7748, -115.6656) -> (-54.2957, -115.6655)
  point P0 (0, 0)
  constraints: 6 end point, 1 perpendicular
extrude "Выдавливание9" cut sketch "Эскиз9" against normal through all contours L176 L175 L174 L173 L183 L182 L181 L184 L185
sketch "Эскиз10" plane through (0, 0, 5) normal (0, 0, 1) x (1, 0, 0)
  line L0 (-46.3063, -82.796) -> (-55.7751, -112.8815) projected
  line L1 (-55.7751, -112.8815) -> (-55.7748, -115.6656) projected
  line L2 (-55.7748, -115.6656) -> (-54.2957, -115.6655) projected
  line L3 (-54.2957, -115.6655) -> (-29.9022, -115.8548) projected
  line L4 (-29.9022, -115.8548) -> (-46.2049, -99.4426) projected
  line L5 (-46.2049, -99.4426) -> (-41.3132, -83.8997) projected
  line L6 (-41.3132, -83.8997) -> (-41.2444, -83.7977) projected
  line L7 (-26.1708, -65.5638) -> (-41.2444, -83.7977) projected
  line L8 (-26.1708, -65.5638) -> (-26.1132, -65.2728) projected
  line L9 (-26.2817, -65.1065) -> (-26.1132, -65.2728) projected
  line L10 (-26.573, -64.8618) -> (-26.2817, -65.1065) projected
  line L11 (-26.8814, -64.6558) -> (-26.573, -64.8618) projected
  line L12 (-27.2145, -64.5081) -> (-26.8814, -64.6558) projected
  line L13 (-27.5361, -64.3327) -> (-27.2145, -64.5081) projected
  line L14 (-27.6899, -64.2282) -> (-27.5361, -64.3327) projected
  line L15 (-27.8382, -64.1096) -> (-27.6899, -64.2282) projected
  line L16 (-27.9796, -63.9735) -> (-27.8382, -64.1096) projected
  line L17 (-28.112, -63.8133) -> (-27.9796, -63.9735) projected
  line L18 (-28.1736, -63.7205) -> (-28.112, -63.8133) projected
  line L19 (-28.2309, -63.6153) -> (-28.1736, -63.7205) projected
  line L20 (-28.2817, -63.4914) -> (-28.2309, -63.6153) projected
  line L21 (-28.3209, -63.3328) -> (-28.2817, -63.4914) projected
  line L22 (-28.2942, -62.9735) -> (-28.3209, -63.3328) projected
  line L23 (-28.085, -62.2597) -> (-28.2942, -62.9735) projected
  line L24 (-27.9195, -61.5344) -> (-28.085, -62.2597) projected
  line L25 (-27.7675, -61.2078) -> (-27.9195, -61.5344) projected
  line L26 (-27.6559, -61.0885) -> (-27.7675, -61.2078) projected
  line L27 (-27.5511, -61.0052) -> (-27.6559, -61.0885) projected
  line L28 (-27.4498, -60.9413) -> (-27.5511, -61.0052) projected
  line L29 (-27.3508, -60.8903) -> (-27.4498, -60.9413) projected
  line L30 (-27.1571, -60.815) -> (-27.3508, -60.8903) projected
  line L31 (-26.9672, -60.7651) -> (-27.1571, -60.815) projected
  line L32 (-26.78, -60.734) -> (-26.9672, -60.7651) projected
  line L33 (-26.5947, -60.7178) -> (-26.78, -60.734) projected
  line L34 (-26.2284, -60.7215) -> (-26.5947, -60.7178) projected
  line L35 (-25.8656, -60.755) -> (-26.2284, -60.7215) projected
  line L36 (-25.4958, -60.7256) -> (-25.8656, -60.755) projected
  line L37 (-25.1221, -60.6541) -> (-25.4958, -60.7256) projected
  line L38 (-24.7463, -60.5502) -> (-25.1221, -60.6541) projected
  line L39 (-24.3693, -60.4182) -> (-24.7463, -60.5502) projected
  line L40 (-23.9923, -60.2602) -> (-24.3693, -60.4182) projected
  line L41 (-23.616, -60.0777) -> (-23.9923, -60.2602) projected
  line L42 (-23.2412, -59.8717) -> (-23.616, -60.0777) projected
  line L43 (-22.8687, -59.6431) -> (-23.2412, -59.8717) projected
  line L44 (-22.4992, -59.3924) -> (-22.8687, -59.6431) projected
  line L45 (-22.2246, -59.1902) -> (-22.4992, -59.3924) projected
  line L46 (-22.3522, -57.0445) -> (-22.2246, -59.1902) projected
  line L47 (-22.6489, -56.8763) -> (-22.3522, -57.0445) projected
  line L48 (-23.0454, -56.6711) -> (-22.6489, -56.8763) projected
  line L49 (-23.4424, -56.4882) -> (-23.0454, -56.6711) projected
  line L50 (-23.839, -56.3281) -> (-23.4424, -56.4882) projected
  line L51 (-24.2343, -56.1915) -> (-23.839, -56.3281) projected
  line L52 (-24.6274, -56.0793) -> (-24.2343, -56.1915) projected
  line L53 (-25.0173, -55.9929) -> (-24.6274, -56.0793) projected
  line L54 (-25.4028, -55.9343) -> (-25.0173, -55.9929) projected
  line L55 (-25.7823, -55.9075) -> (-25.4028, -55.9343) projected
  line L56 (-26.153, -55.9222) -> (-25.7823, -55.9075) projected
  line L57 (-26.5093, -55.9985) -> (-26.153, -55.9222) projected
  line L58 (-26.8725, -56.0456) -> (-26.5093, -55.9985) projected
  line L59 (-27.0584, -56.0515) -> (-26.8725, -56.0456) projected
  line L60 (-27.248, -56.0427) -> (-27.0584, -56.0515) projected
  line L61 (-27.4425, -56.0157) -> (-27.248, -56.0427) projected
  line L62 (-27.6437, -55.9639) -> (-27.4425, -56.0157) projected
  line L63 (-27.7481, -55.925) -> (-27.6437, -55.9639) projected
  line L64 (-27.8563, -55.8736) -> (-27.7481, -55.925) projected
  line L65 (-27.9702, -55.8032) -> (-27.8563, -55.8736) projected
  line L66 (-28.0951, -55.698) -> (-27.9702, -55.8032) projected
  line L67 (-28.2847, -55.3917) -> (-28.0951, -55.698) projected
  line L68 (-28.5351, -54.6912) -> (-28.2847, -55.3917) projected
  line L69 (-28.8274, -54.0071) -> (-28.5351, -54.6912) projected
  line L70 (-28.8965, -53.6536) -> (-28.8274, -54.0071) projected
  line L71 (-28.8763, -53.4914) -> (-28.8965, -53.6536) projected
  line L72 (-28.8405, -53.3624) -> (-28.8763, -53.4914) projected
  line L73 (-28.7962, -53.2512) -> (-28.8405, -53.3624) projected
  line L74 (-28.746, -53.1517) -> (-28.7962, -53.2512) projected
  line L75 (-28.6335, -52.977) -> (-28.746, -53.1517) projected
  line L76 (-28.5092, -52.825) -> (-28.6335, -52.977) projected
  line L77 (-28.3761, -52.6897) -> (-28.5092, -52.825) projected
  line L78 (-28.2357, -52.5677) -> (-28.3761, -52.6897) projected
  line L79 (-27.9372, -52.3554) -> (-28.2357, -52.5677) projected
  line L80 (-27.624, -52.1693) -> (-27.9372, -52.3554) projected
  line L81 (-27.3421, -51.9282) -> (-27.624, -52.1693) projected
  line L82 (-27.0818, -51.6507) -> (-27.3421, -51.9282) projected
  line L83 (-26.8388, -51.3457) -> (-27.0818, -51.6507) projected
  line L84 (-26.6114, -51.0173) -> (-26.8388, -51.3457) projected
  line L85 (-26.3993, -50.6679) -> (-26.6114, -51.0173) projected
  line L86 (-26.2021, -50.2991) -> (-26.3993, -50.6679) projected
  line L87 (-26.02, -49.9121) -> (-26.2021, -50.2991) projected
  line L88 (-25.853, -49.5082) -> (-26.02, -49.9121) projected
  line L89 (-25.7014, -49.0882) -> (-25.853, -49.5082) projected
  line L90 (-25.5981, -48.7632) -> (-25.7014, -49.0882) projected
  line L91 (-25.5981, -48.7632) -> (-26.9625, -47.1023) projected
  line L92 (-27.3014, -47.1406) -> (-26.9625, -47.1023) projected
  line L93 (-27.7429, -47.2077) -> (-27.3014, -47.1406) projected
  line L94 (-28.1715, -47.2931) -> (-27.7429, -47.2077) projected
  line L95 (-28.5864, -47.3967) -> (-28.1715, -47.2931) projected
  line L96 (-28.9865, -47.5185) -> (-28.5864, -47.3967) projected
  line L97 (-29.3705, -47.6588) -> (-28.9865, -47.5185) projected
  line L98 (-29.7368, -47.818) -> (-29.3705, -47.6588) projected
  line L99 (-30.0831, -47.9973) -> (-29.7368, -47.818) projected
  line L100 (-30.4059, -48.1987) -> (-30.0831, -47.9973) projected
  line L101 (-30.6971, -48.4284) -> (-30.4059, -48.1987) projected
  line L102 (-30.9405, -48.6995) -> (-30.6971, -48.4284) projected
  line L103 (-31.2067, -48.9511) -> (-30.9405, -48.6995) projected
  line L104 (-31.3536, -49.0652) -> (-31.2067, -48.9511) projected
  line L105 (-31.5122, -49.1695) -> (-31.3536, -49.0652) projected
  line L106 (-31.6854, -49.262) -> (-31.5122, -49.1695) projected
  line L107 (-31.8786, -49.3384) -> (-31.6854, -49.262) projected
  line L108 (-31.986, -49.3683) -> (-31.8786, -49.3384) projected
  line L109 (-32.1037, -49.3902) -> (-31.986, -49.3683) projected
  line L110 (-32.2372, -49.4003) -> (-32.1037, -49.3902) projected
  line L111 (-32.4002, -49.3886) -> (-32.2372, -49.4003) projected
  line L112 (-32.7336, -49.2522) -> (-32.4002, -49.3886) projected
  line L113 (-33.3479, -48.8326) -> (-32.7336, -49.2522) projected
  line L114 (-33.9864, -48.4511) -> (-33.3479, -48.8326) projected
  line L115 (-34.2501, -48.2056) -> (-33.9864, -48.4511) projected
  line L116 (-34.3291, -48.0626) -> (-34.2501, -48.2056) projected
  line L117 (-34.376, -47.9372) -> (-34.3291, -48.0626) projected
  line L118 (-34.4055, -47.8211) -> (-34.376, -47.9372) projected
  line L119 (-34.4234, -47.7112) -> (-34.4055, -47.8211) projected
  line L120 (-34.4351, -47.5037) -> (-34.4234, -47.7112) projected
  line L121 (-34.4238, -47.3077) -> (-34.4351, -47.5037) projected
  line L122 (-34.3956, -47.12) -> (-34.4238, -47.3077) projected
  line L123 (-34.3538, -46.9387) -> (-34.3956, -47.12) projected
  line L124 (-34.237, -46.5916) -> (-34.3538, -46.9387) projected
  line L125 (-34.0931, -46.2568) -> (-34.237, -46.5916) projected
  line L126 (-34.0067, -45.8961) -> (-34.0931, -46.2568) projected
  line L127 (-33.9593, -45.5186) -> (-34.0067, -45.8961) projected
  line L128 (-33.9419, -45.129) -> (-33.9593, -45.5186) projected
  line L129 (-33.951, -44.7298) -> (-33.9419, -45.129) projected
  line L130 (-33.9848, -44.3224) -> (-33.951, -44.7298) projected
  line L131 (-34.0421, -43.9081) -> (-33.9848, -44.3224) projected
  line L132 (-34.1221, -43.488) -> (-34.0421, -43.9081) projected
  line L133 (-34.2244, -43.063) -> (-34.1221, -43.488) projected
  line L134 (-34.3487, -42.6342) -> (-34.2244, -43.063) projected
  line L135 (-34.4561, -42.3105) -> (-34.3487, -42.6342) projected
  line L136 (-36.5363, -41.7688) -> (-34.4561, -42.3105) projected
  line L137 (-36.7879, -41.999) -> (-36.5363, -41.7688) projected
  line L138 (-37.1056, -42.3127) -> (-36.7879, -41.999) projected
  line L139 (-37.4022, -42.6338) -> (-37.1056, -42.3127) projected
  line L140 (-37.677, -42.9614) -> (-37.4022, -42.6338) projected
  line L141 (-37.9291, -43.2952) -> (-37.677, -42.9614) projected
  line L142 (-38.1573, -43.6344) -> (-37.9291, -43.2952) projected
  line L143 (-38.36, -43.9785) -> (-38.1573, -43.6344) projected
  line L144 (-38.5348, -44.327) -> (-38.36, -43.9785) projected
  line L145 (-38.6775, -44.6797) -> (-38.5348, -44.327) projected
  line L146 (-38.7781, -45.0367) -> (-38.6775, -44.6797) projected
  line L147 (-38.8157, -45.3992) -> (-38.7781, -45.0367) projected
  line L148 (-38.8831, -45.7592) -> (-38.8157, -45.3992) projected
  line L149 (-38.935, -45.9378) -> (-38.8831, -45.7592) projected
  line L150 (-39.0019, -46.1155) -> (-38.935, -45.9378) projected
  line L151 (-39.0877, -46.292) -> (-39.0019, -46.1155) projected
  line L152 (-39.1991, -46.4674) -> (-39.0877, -46.292) projected
  line L153 (-39.2684, -46.5547) -> (-39.1991, -46.4674) projected
  line L154 (-39.3507, -46.6417) -> (-39.2684, -46.5547) projected
  line L155 (-39.4528, -46.7283) -> (-39.3507, -46.6417) projected
  line L156 (-39.5916, -46.8146) -> (-39.4528, -46.7283) projected
  line L157 (-39.9414, -46.9002) -> (-39.5916, -46.8146) projected
  line L158 (-40.685, -46.9219) -> (-39.9414, -46.9002) projected
  line L159 (-41.4259, -46.9885) -> (-40.685, -46.9219) projected
  line L160 (-41.7835, -46.9449) -> (-41.4259, -46.9885) projected
  line L161 (-41.9315, -46.8757) -> (-41.7835, -46.9449) projected
  line L162 (-42.0431, -46.8018) -> (-41.9315, -46.8757) projected
  line L163 (-42.1352, -46.7252) -> (-42.0431, -46.8018) projected
  line L164 (-42.2143, -46.6467) -> (-42.1352, -46.7252) projected
  line L165 (-42.3457, -46.4857) -> (-42.2143, -46.6467) projected
  line L166 (-42.4518, -46.3206) -> (-42.3457, -46.4857) projected
  line L167 (-42.5394, -46.1522) -> (-42.4518, -46.3206) projected
  line L168 (-42.612, -45.9809) -> (-42.5394, -46.1522) projected
  line L169 (-42.7217, -45.6314) -> (-42.612, -45.9809) projected
  line L170 (-42.8019, -45.276) -> (-42.7217, -45.6314) projected
  line L171 (-42.9441, -44.9334) -> (-42.8019, -45.276) projected
  line L172 (-43.1276, -44.6002) -> (-42.9441, -44.9334) projected
  line L173 (-43.3425, -44.2748) -> (-43.1276, -44.6002) projected
  line L174 (-43.5846, -43.9571) -> (-43.3425, -44.2748) projected
  line L175 (-43.8514, -43.6473) -> (-43.5846, -43.9571) projected
  line L176 (-44.1412, -43.3458) -> (-43.8514, -43.6473) projected
  line L177 (-44.4529, -43.053) -> (-44.1412, -43.3458) projected
  line L178 (-44.5941, -42.9326) -> (-44.4529, -43.053) projected
  arc A0 (-44.5941, -42.9326) -> (-50.5827, -73.1948) centre (-31.1137, -61.3239) ccw projected
  arc A1 (-46.3063, -82.796) -> (-50.5827, -73.1948) centre (-85.5886, -94.5392) ccw projected
  circle A2 centre (-42.8052, -51.6922) radius 1.6 projected
  circle A3 centre (-39.9568, -59.168) radius 2.5 projected
  circle A4 centre (-32.4811, -56.3196) radius 1.6 projected
  circle A5 centre (-37.1084, -66.6437) radius 1.6 projected
  circle A6 centre (-47.4326, -62.0164) radius 1.6 projected
  circle A7 centre (-39.9568, -59.168) radius 12.2678
  point P0 (0, 0)
  point P1 (-41.4259, -46.9885)
  constraints: 1 coincident, 3 other
extrude "Выдавливание10" cut sketch "Эскиз10" against normal through all contours A1 A0 L178 L177 L176 L175 L174 L173 L172 L171 L170 L169 L168 L167 L166 L165 L164 L163 L162 L161 L160 A7 L22 L21 L20 L19 L18 L17 L16 L15 L14 L13 L12 L11 L10 L9 L8 L7 L6 L5 L4 L3 L2 L1 L0